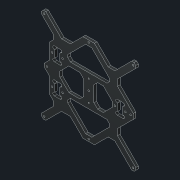
# Autodesk Inventor part: MINI-y-carriage
Saved by Autodesk Inventor 2021 (Build 250183000, 183)
## iProperties
Company: Prusa Development a.s.
Created: 2019-07-16
Material: Všeobecné
Document SubType Name: Modeling
Density: 1 g/cm^3
Appearance: Železo – šedé
Mass: 61.0324 g
Surface Area: 344.548 cm^2
Volume: 61.0324 cm^3
Project: ORIGINAL PRUSA MINI
Authority: Ing. Robert Turinský
Author: Ing. Robert Turinský
Title: MINI-y-carriage
Revision Number: R4
## iProperties of the stored document _3DPrint.ipt
Created: 2021-05-16
Part Number: _3DPrint
Material: Generic
Document SubType Name: Modeling
Designer: arbra
Density: 1 g/cm^3
Appearance: Default
Author: arbra
Autodesk Inventor part; units mm, degrees
ref_plane "YZ Plane" through (0, 0, 0) normal (1, 0, 0) x (0, 1, 0)
sketch "Náčrt1" plane through (0, 0, 0) normal (0, 0, 1) x (1, 0, 0)
  line L0 (0, -126) -> (0, 126) projected
  line L1 (-126, 0) -> (126, 0) projected
  line L2 (-11, 84) -> (11, 84)
  line L3 (11, 84) -> (37, 58)
  line L4 (37, 58) -> (50, 58)
  line L5 (50, 58) -> (82, 90)
  line L6 (90, 82) -> (55, 47)
  line L7 (55, 47) -> (55, 35)
  line L8 (55, 35) -> (85, 5)
  line L9 (85, 5) -> (85, -5)
  circle A0 centre (85, 85) radius 1.6
  line L10 (86.7767, 90) -> (90, 86.7767)
  line L11 (82, 90) -> (86.7767, 90)
  line L12 (90, 86.7767) -> (90, 82)
  line L13 (-11, 84) -> (-35, 60)
  line L14 (-35, 60) -> (-52, 60)
  line L15 (-52, 60) -> (-82, 90)
  line L16 (-82, 90) -> (-86.7767, 90)
  line L17 (-86.7767, 90) -> (-90, 86.7767)
  line L18 (-90, 86.7767) -> (-90, 82)
  line L19 (-90, 82) -> (-68, 60)
  line L20 (-68, 60) -> (-68, 50)
  circle A1 centre (-85, 85) radius 1.6
  line L21 (-68, 50) -> (-75, 43)
  line L22 (-75, 43) -> (-75, 13)
  line L23 (-75, 13) -> (-85, 3)
  line L24 (-85, 3) -> (-85, -3)
  line L25 (-6, 74) -> (6, 74)
  line L26 (6, 74) -> (40, 40)
  line L27 (40, 40) -> (40, 35)
  line L28 (40, 35) -> (35, 30)
  line L29 (35, 30) -> (-35, 30)
  line L30 (-35, 30) -> (-40, 35)
  line L31 (-40, 35) -> (-40, 40)
  line L32 (-40, 40) -> (-6, 74)
  circle A2 centre (0, 80) radius 1.6
  line L33 (-10, -15) -> (-10, 15)
  line L34 (-10, 15) -> (-17, 22)
  line L35 (-17, 22) -> (-38, 22)
  line L36 (-38, 22) -> (-55, 5)
  line L37 (-55, 5) -> (-55, -5)
  line L38 (10, -15) -> (10, 15)
  line L39 (10, 15) -> (17, 22)
  line L40 (17, 22) -> (28, 22)
  line L41 (28, 22) -> (45, 5)
  line L42 (45, 5) -> (45, -5)
  circle A3 centre (0, 20) radius 1.25
  circle A4 centre (0, 0) radius 1.6
  line L43 (-65, 35) -> (-65, 21.5)
  line L44 (-55, 35) -> (-55, 21.5)
  line L45 (-65.5, 41.5) -> (-54.5, 41.5)
  arc A5 (-65.5, 41.5) -> (-65.5, 35.5) centre (-65.5, 38.5) ccw
  arc A6 (-54.5, 35.5) -> (-54.5, 41.5) centre (-54.5, 38.5) ccw
  line L46 (-65.5, 35.5) -> (-65, 35)
  line L47 (-54.5, 35.5) -> (-55, 35)
  line L48 (-65, 21.5) -> (-65.5, 21)
  line L49 (-55, 21.5) -> (-54.5, 21)
  line L50 (-65.5, 15) -> (-54.5, 15)
  arc A7 (-65.5, 21) -> (-65.5, 15) centre (-65.5, 18) ccw
  arc A8 (-54.5, 15) -> (-54.5, 21) centre (-54.5, 18) ccw
  circle A9 centre (-70, 28.25) radius 1.6
  circle A10 centre (-50, 28.25) radius 1.6
  line L51 (-60, 41.5) -> (-60, 37.7564)
  line L52 (55, 6.75) -> (55, -6.75)
  line L53 (65, 6.75) -> (65, -6.75)
  line L54 (54.5, 13.25) -> (65.5, 13.25)
  arc A11 (54.5, 13.25) -> (54.5, 7.25) centre (54.5, 10.25) ccw
  arc A12 (65.5, 7.25) -> (65.5, 13.25) centre (65.5, 10.25) ccw
  line L55 (54.5, 7.25) -> (55, 6.75)
  line L56 (65.5, 7.25) -> (65, 6.75)
  line L57 (55, -6.75) -> (54.5, -7.25)
  line L58 (65, -6.75) -> (65.5, -7.25)
  line L59 (54.5, -13.25) -> (65.5, -13.25)
  arc A13 (54.5, -7.25) -> (54.5, -13.25) centre (54.5, -10.25) ccw
  arc A14 (65.5, -13.25) -> (65.5, -7.25) centre (65.5, -10.25) ccw
  circle A15 centre (50, 0) radius 1.6
  circle A16 centre (70, 0) radius 1.6
  line L60 (60, 13.25) -> (60, 9.5064)
  circle A17 centre (-80, 0) radius 1.6
  circle A18 centre (80, 0) radius 1.6
  line L61 (-11, -84) -> (11, -84)
  line L62 (11, -84) -> (37, -58)
  line L63 (37, -58) -> (50, -58)
  line L64 (50, -58) -> (82, -90)
  line L65 (90, -82) -> (55, -47)
  line L66 (55, -47) -> (55, -35)
  line L67 (55, -35) -> (85, -5)
  circle A19 centre (85, -85) radius 1.6
  line L68 (86.7767, -90) -> (90, -86.7767)
  line L69 (82, -90) -> (86.7767, -90)
  line L70 (90, -86.7767) -> (90, -82)
  line L71 (-11, -84) -> (-35, -60)
  line L72 (-35, -60) -> (-52, -60)
  line L73 (-52, -60) -> (-82, -90)
  line L74 (-82, -90) -> (-86.7767, -90)
  line L75 (-86.7767, -90) -> (-90, -86.7767)
  line L76 (-90, -86.7767) -> (-90, -82)
  line L77 (-90, -82) -> (-68, -60)
  line L78 (-68, -60) -> (-68, -50)
  circle A20 centre (-85, -85) radius 1.6
  line L79 (-68, -50) -> (-75, -43)
  line L80 (-75, -43) -> (-75, -13)
  line L81 (-75, -13) -> (-85, -3)
  line L82 (-6, -74) -> (6, -74)
  line L83 (6, -74) -> (40, -40)
  line L84 (40, -40) -> (40, -35)
  line L85 (40, -35) -> (35, -30)
  line L86 (35, -30) -> (-35, -30)
  line L87 (-35, -30) -> (-40, -35)
  line L88 (-40, -35) -> (-40, -40)
  line L89 (-40, -40) -> (-6, -74)
  circle A21 centre (0, -80) radius 1.6
  line L90 (-10, -15) -> (-17, -22)
  line L91 (-17, -22) -> (-38, -22)
  line L92 (-38, -22) -> (-55, -5)
  line L93 (10, -15) -> (17, -22)
  line L94 (17, -22) -> (28, -22)
  line L95 (28, -22) -> (45, -5)
  circle A22 centre (0, -20) radius 1.25
  line L96 (-65, -35) -> (-65, -21.5)
  line L97 (-55, -35) -> (-55, -21.5)
  line L98 (-65.5, -41.5) -> (-54.5, -41.5)
  arc A23 (-65.5, -35.5) -> (-65.5, -41.5) centre (-65.5, -38.5) ccw
  arc A24 (-54.5, -41.5) -> (-54.5, -35.5) centre (-54.5, -38.5) ccw
  line L99 (-65.5, -35.5) -> (-65, -35)
  line L100 (-54.5, -35.5) -> (-55, -35)
  line L101 (-65, -21.5) -> (-65.5, -21)
  line L102 (-55, -21.5) -> (-54.5, -21)
  arc A25 (-65.5, -15) -> (-65.5, -21) centre (-65.5, -18) ccw
  arc A26 (-54.5, -21) -> (-54.5, -15) centre (-54.5, -18) ccw
  circle A27 centre (-70, -28.25) radius 1.6
  circle A28 centre (-50, -28.25) radius 1.6
  line L103 (-60, -41.5) -> (-60, -37.7564)
  line L104 (-65.5, -15) -> (-54.5, -15)
  circle A29 centre (-70, 28.25) radius 1.6
  circle A30 centre (-50, 28.25) radius 1.6
  circle A31 centre (50, 0) radius 1.6
  circle A32 centre (70, 0) radius 1.6
  circle A33 centre (-70, -28.25) radius 1.6
  circle A34 centre (-50, -28.25) radius 1.6
  point P0 (-10, 0)
  point P1 (10, 0)
  point P2 (-55, 28.25)
  point P3 (65, 0)
  point P4 (-55, -28.25)
  dimension "d0" = 84
  dimension "d1" = 85
  dimension "d2" = 85
  dimension "d5" = 45
  dimension "d6" = 3.2
  dimension "d8" = 90
  dimension "d9" = 90
  dimension "d11" = 125
  dimension "d13" = 22
  dimension "d14" = 13
  dimension "d15" = 12
  dimension "d16" = 10
  dimension "d17" = 17
  dimension "d19" = 7
  dimension "d20" = 10
  dimension "d21" = 6
  dimension "d22" = 80
  dimension "d23" = 44
  dimension "d24" = 5
  dimension "d25" = 10
  dimension "d26" = 80
  dimension "d27" = 17
  dimension "d28" = 7
  dimension "d29" = 10
  dimension "d30" = 45
  dimension "d31" = 22
  dimension "d32" = 35
  dimension "d33" = 20
  dimension "d34" = 10
  dimension "d35" = 0.5
  dimension "d36" = 3
  dimension "d37" = 26.5
  dimension "d38" = 20
  dimension "d39" = 55
  dimension "d40" = 28.25
  dimension "d41" = 10
  dimension "d42" = 0.5
  dimension "d43" = 3
  dimension "d44" = 26.5
  dimension "d45" = 20
  dimension "d46" = 55
  dimension "d47" = 80
  dimension "d53" = 3.2
  dimension "d76" = 2.5
  dimension "d77" = 82
  dimension "d78" = 82
  constraints: 206 end point, 74 symmetric about line, 35 centre point, 26 perpendicular, 24 point on circle, 20 equal radius, 10 parallel, 10 vertical alignment, 8 horizontal, 8 point on line, 8 tangent, 8 vertical, 6 equal length, 6 midpoint, 5 horizontal alignment, 1 coincident, 1 collinear, 19 other
  measures "d0" distance between parallel lines of L1 L2
  measures "d1" distance from line of L0 A0.centre
  measures "d2" distance from line of L1 A0.centre
  measures "d5" angle of L3 L0
  measures "d6" diameter of A0
  measures "d8" distance between parallel lines of L0 L12
  measures "d9" distance between parallel lines of L1 L11
  measures "d11" distance from line of L10 point (0, 0)
  measures "d13" distance of L2.start L2.end
  measures "d14" distance of L3.end L4.end
  measures "d15" distance of L6.end L7.end
  measures "d16" distance of L8.end L9.end
  measures "d17" distance of L13.end L14.end
  measures "d19" distance between parallel lines of L20 L22
  measures "d20" distance between parallel lines of L22 L24
  measures "d21" distance of L23.end L24.end
  measures "d22" distance between parallel lines of L27 L31
  measures "d23" distance between parallel lines of L29 L25
  measures "d24" horizontal distance of L27.end L28.end
  measures "d25" distance between parallel lines of L2 L25
  measures "d26" distance from line of L1 A2.centre
  measures "d27" horizontal distance of L35.end L36.end
  measures "d28" horizontal distance of L33.end L34.end
  measures "d29" distance between parallel lines of L0 L33
  measures "d30" distance between parallel lines of L33 L37
  measures "d31" distance between parallel lines of L1 L35
  measures "d32" distance between parallel lines of L38 L42
  measures "d33" distance of A4.centre A3.centre
  measures "d34" distance between parallel lines of L44 L43
  measures "d35" horizontal distance of L47.start L44.start
  measures "d36" radius of A6
  measures "d37" distance between parallel lines of L50 L45
  measures "d38" distance of A10.centre A9.centre
  measures "d39" distance between parallel lines of L0 L44
  measures "d40" distance from line of L1 A9.centre
  measures "d41" distance between parallel lines of L53 L52
  measures "d42" horizontal distance of L56.start L56.end
  measures "d43" radius of A12
  measures "d44" distance between parallel lines of L59 L54
  measures "d45" distance of A16.centre A15.centre
  measures "d46" distance between parallel lines of L0 L52
  measures "d47" distance from line of L0 A17.centre
  measures "d53" diameter of A29
  measures "d76" diameter of A3
  measures "d77" distance from line of L0 L5.end
  measures "d78" distance from line of L1 L6.start
extrude "Vysunutí1" add sketch "Náčrt1" along normal blind 5 contours L61 L71 L72 L73 L74 L75 L76 L77 L78 L79 L80 L81 L24 L1 A17 L37 L92 L91 L90 L33 A4 L0 A22 L86 L87 L88 L89 L82 A21 | L0 A21 L82 L83 L84 L85 L86 A22 A4 L1 L38 L93 L94 L95 L42 A15 L52 L57 A13 L59 A14 L58 L53 A16 A18 L9 L67 L66 L65 L70 L68 L69 L64 L63 L62 L61 | L1 L33 L34 L35 L36 L37 A17 L24 L23 L22 L21 L20 L19 L18 L17 L16 L15 L14 L13 L2 L0 A2 L25 L32 L31 L30 L29 A3 A4 | A4 L0 A3 L29 L28 L27 L26 L25 A2 L2 L3 L4 L5 L11 L10 L12 L6 L7 L8 L9 L1 A18 A16 L53 L56 A12 L54 A11 L55 L52 A15 L42 L41 L40 L39 L38
sketch "Náčrt2" plane through (0, 0, 0) normal (0, 1, 0) x (-1, 0, 0)
  circle A0 centre (-60, -5.5902) radius 7.5
  circle A1 centre (60, -5.5902) radius 7.5
  point P0 (0, 0)
  point P1 (55, 0)
  point P2 (65, 0)
  point P3 (-55, 0)
  point P4 (-65, 0)
  dimension "d50" = 15
  constraints: 4 point on circle, 2 centre point, 1 equal radius
  measures "d50" diameter of A0
ref_plane "Pracovní rovina1" through (0, 28.25, 0) normal (0, 1, 0) x (-1, 0, 0)
ref_plane "Pracovní rovina2" through (0, -28.25, 0) normal (0, 1, 0) x (-1, 0, 0)
thread "Závit1" size "M3x0.5" class "6H" standard "ANSI Metric M Profile" full length
thread "Závit2" size "M3x0.5" class "6H" standard "ANSI Metric M Profile" full length
thread "Závit3" size "M3x0.5" class "6H" standard "ANSI Metric M Profile" full length
thread "Závit4" size "M3x0.5" class "6H" standard "ANSI Metric M Profile" full length
thread "Závit5" size "M3x0.5" class "6H" standard "ANSI Metric M Profile" full length
thread "Závit6" size "M3x0.5" class "6H" standard "ANSI Metric M Profile" full length
thread "Závit7" size "M3x0.5" class "6H" standard "ANSI Metric M Profile" full length
thread "Závit8" size "M3x0.5" class "6H" standard "ANSI Metric M Profile" full length
thread "Závit9" size "M3x0.5" class "6H" standard "ANSI Metric M Profile" full length
thread "Závit10" size "M3x0.5" class "6H" standard "ANSI Metric M Profile" full length
thread "Závit11" size "M3x0.5" class "6H" standard "ANSI Metric M Profile" full length
equation "\"d2\" = d1"
equation "\"d9\" = d8"
equation "\"d46\" = d39"
